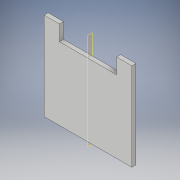
# Autodesk Inventor part: plate
Saved by Autodesk Inventor 2019.3 (Build 233278000, 278)
## iProperties
Created: 2019-06-11
Part Number: plate
Material: Generic
Document SubType Name: Modeling
Designer: Frienddo
Density: 1 g/cm^3
Appearance: Default
Author: Frienddo
Autodesk Inventor part; units mm, degrees
ref_plane "XZ Plane" through (0, 0, 0) normal (0, 1, 0) x (-1, 0, 0)
ref_plane "XY Plane" through (0, 0, 0) normal (0, 0, 1) x (1, 0, 0)
sketch "Sketch1" plane through (0, 0, 0) normal (0, 0, 1) x (1, 0, 0)
  line L0 (43, -43) -> (-43, -43)
  line L1 (-43, -43) -> (-43, 43)
  line L2 (-43, 43) -> (43, 43)
  line L3 (43, 43) -> (43, -43)
  line L4 (43, -43) -> (-43, 43) construction
  line L5 (-43, -43) -> (43, 43) construction
  line L6 (-28, 43) -> (28, 43)
  line L7 (28, 43) -> (28, 28)
  line L8 (28, 28) -> (-28, 28)
  line L9 (-28, 28) -> (-28, 43)
  line L10 (-33, -43) -> (37, -43)
  line L11 (0, 60.2) -> (0, -60.2) projected
  point P0 (0, 0)
  dimension "d0" = 86
  dimension "d1" = 86
  dimension "d2" = 15
  constraints: 22 end point, 4 parallel, 4 point on line, 3 horizontal, 2 midpoint, 2 perpendicular
  measures "d0" distance of L1.end L2.end
  measures "d1" distance of L0.end L1.end
  measures "d2" distance of L6.end L7.end
extrude "Extrusion1" add sketch "Sketch1" along normal blind 4 contours L0 L11 L8 L7 L2 L3 | L0 L1 L2 L9 L8 L11
body "Solid1"
